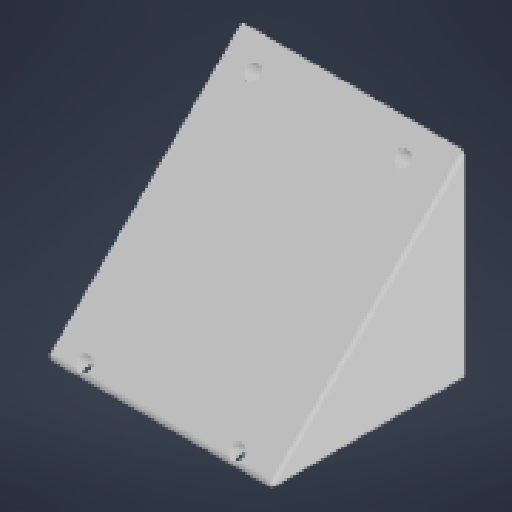
# Autodesk Inventor part: Part16
Saved by Autodesk Inventor 2026.2 (Build 302298000, 298)
## iProperties
Created: 2026-05-30
Part Number: Part16
Material: Generic
Document SubType Name: Modeling
Designer: FromDarkHell
Density: 1 g/cm^3
Appearance: Default
Author: FromDarkHell
Autodesk Inventor part; units mm, degrees
ref_plane "YZ Plane" through (0, 0, 0) normal (1, 0, 0) x (0, 1, 0)
ref_plane "XZ Plane" through (0, 0, 0) normal (0, 1, 0) x (-1, 0, 0)
ref_plane "XY Plane" through (0, 0, 0) normal (0, 0, 1) x (1, 0, 0)
sketch "Sketch2" plane through (0, 0, 0) normal (1, 0, 0) x (0, 1, 0)
  line L0 (-7.5199, -16.943) -> (37.3814, -61.8443)
  line L1 (37.3814, -61.8443) -> (-7.5199, -61.8443)
  line L2 (-7.5199, -16.943) -> (-7.5199, -61.8443)
  point P0 (0, 0)
  dimension "d0" = 63.5
  dimension "d3" = 45
  constraints: 6 end point, 1 horizontal, 1 vertical
  measures "d0" distance of L0.start L0.end
  measures "d3" angle of L0 L1
extrude "Extrusion1" add sketch "Sketch2" along normal blind 50.8
sketch "Sketch4" plane through (0, -7.5199, -16.943) normal (0, 0.7071, 0.7071) x (1, 0, 0)
  circle A0 centre (41.65, 3.675) radius 1.6 projected
  circle A1 centre (41.15, 57.425) radius 1.6 projected
  circle A2 centre (7.15, 57.425) radius 1.6 projected
  circle A3 centre (7.15, 3.675) radius 1.6 projected
  point P0 (0, -6.6631)
extrude "Extrusion3" cut sketch "Sketch4" against normal through all
fillet "Fillet1" radius 1 4 edges at (50.8, -7.5199, -39.3936) (50.8, 14.9307, -39.3936) (0, 14.9307, -39.3936) (0, -7.5199, -39.3936)
body "Solid1"
